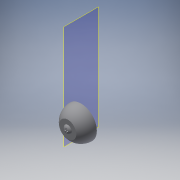
# Autodesk Inventor part: Part44
Saved by Autodesk Inventor 2016 (Build 200138000, 138)
## iProperties
Created: 2016-01-27
Part Number: Part44
Material: Generic
Document SubType Name: Modeling
Designer: seve
Density: 1 g/cm^3
Appearance: Default
Author: seve
Autodesk Inventor part; units mm, degrees
ref_plane "YZ Plane" through (0, 0, 0) normal (1, 0, 0) x (0, 1, 0)
ref_plane "XZ Plane" through (0, 0, 0) normal (0, 1, 0) x (-1, 0, 0)
ref_plane "XY Plane" through (0, 0, 0) normal (0, 0, 1) x (1, 0, 0)
sketch "Sketch2" plane through (0, 0, 0) normal (0, 0, 1) x (1, 0, 0)
  circle A0 centre (0, -1.463003) radius 3.175
  point P0 (0, 0)
  dimension "d2" = 6.35
  constraints: 1 centre point
  measures "d2" diameter of A0
extrude "Extrusion2" add sketch "Sketch2" along normal blind 3.175
fillet "Fillet1" radius 3.175 1 edges at (-3.175, -1.463, 3.175)
ref_plane "Work Plane1" through (-3.175, 6.35, -6.35) normal (-1, 0, 0) x (0, -1, 0)
sketch "Sketch3" plane through (-3.175, 6.35, -6.35) normal (-1, 0, 0) x (0, -1, 0)
  arc A0 (10.988003, 6.35) -> (4.638003, 6.35) centre (7.813003, 6.35) ccw
  line L0 (5.908769, 10.030273) -> (9.516449, 10.030273)
  line L1 (9.516449, 10.030273) -> (9.516449, 9.029346)
  line L2 (9.516449, 9.029346) -> (5.908769, 9.029346)
  line L3 (5.908769, 9.029346) -> (5.908769, 10.030273)
  point P0 (6.35, 6.35)
  constraints: 8 end point, 2 parallel, 1 horizontal, 1 perpendicular, 1 point on circle
extrude "Extrusion3" cut sketch "Sketch3" against normal blind 12.7
sketch "Sketch4" plane through (0, -1.463003, 2.679346) normal (0, 0, 1) x (1, 0, 0)
  circle A0 centre (0, 0) radius 1.703446
  circle A1 centre (0, 0) radius 0.79375
  point P0 (0, 1.463003)
  dimension "d8" = 1.5875
  constraints: 1 centre point, 1 coincident
  measures "d8" diameter of A1
extrude "Extrusion4" add sketch "Sketch4" along normal blind 0.396875 contours A1
fillet "Fillet2" radius 0.79375 1 edges at (-0.7937, -1.463, 3.0762)
sketch "Sketch5" plane through (0, -1.463003, 3.076221) normal (0, 0, 1) x (1, 0, 0)
  line L0 (-0.093723, 0.395508) -> (0.096901, 0.395508)
  line L1 (0.096901, 0.395508) -> (0.096901, -0.398758)
  line L2 (0.096901, -0.398758) -> (-0.093723, -0.398758)
  line L3 (-0.093723, -0.398758) -> (-0.093723, 0.395508)
  line L4 (0.386014, 0.093687) -> (-0.386014, 0.093687)
  line L5 (-0.386014, 0.093687) -> (-0.386014, -0.115999)
  line L6 (-0.386014, -0.115999) -> (0.386014, -0.115999)
  line L7 (0.386014, -0.115999) -> (0.386014, 0.093687)
  point P0 (0, 1.463003)
  constraints: 16 end point, 4 parallel, 2 horizontal, 2 perpendicular
extrude "Extrusion5" cut sketch "Sketch5" against normal blind 0.198437
body "Solid2"
